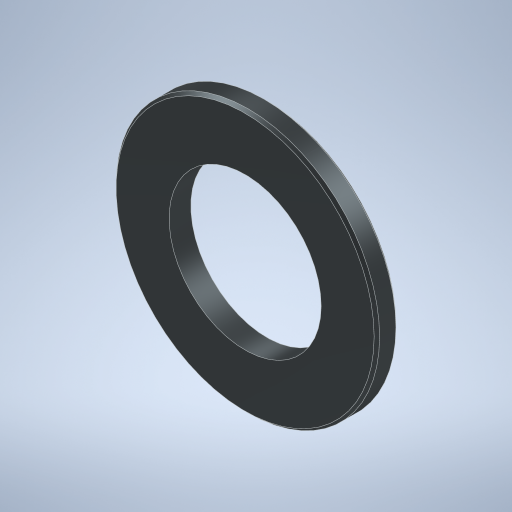
# Autodesk Inventor part: washer_M5
Saved by Autodesk Inventor 2024 (Build 280153000, 153)
## iProperties
Created: 2025-06-10
Part Number: washer_M5
Material: 鉄、ねずみ鋳鉄
Document SubType Name: Modeling
Designer: 1412z
Density: 7.15 g/cm^3
Appearance: 鉄 ねずみ鋳鉄
Author: 1412z
Autodesk Inventor part; units mm, degrees
ref_plane "YZ Plane" through (0, 0, 0) normal (1, 0, 0) x (0, 1, 0)
ref_plane "XZ Plane" through (0, 0, 0) normal (0, 1, 0) x (-1, 0, 0)
ref_plane "XY Plane" through (0, 0, 0) normal (0, 0, 1) x (1, 0, 0)
sketch "スケッチ1" plane through (0, 0, 0) normal (0, 0, 1) x (1, 0, 0)
  circle A0 centre (0, 0) radius 4.85
  circle A1 centre (0, 0) radius 2.8
  dimension "d0" = 9.7
  dimension "d1" = 5.6
  constraints: 2 centre point, 2 coincident
  measures "d0" diameter of A0
  measures "d1" diameter of A1
extrude "押し出し1" add sketch "スケッチ1" along normal blind 0.8
chamfer "面取り1" distance 0.1 angle 45 2 edges at (-4.85, 0, 0.8) (-4.85, 0, 0)
